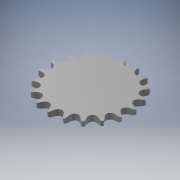
# Autodesk Inventor part: Kettenrad der Rollenkette1
Saved by Autodesk Inventor 2018 (Build 220112000, 112)
## iProperties
Created: 2018-01-11
Part Number: Kettenrad der Rollenkette1
Material: Steel
Document SubType Name: Modeling
Designer: Dominik
Density: 1 g/cm^3
Appearance: Steel
CustomPartVersion: 1
Author: Dominik
Autodesk Inventor part; units mm, degrees
ref_plane "YZ Plane" through (0, 0, 0) normal (1, 0, 0) x (0, 1, 0)
ref_plane "XZ Plane" through (0, 0, 0) normal (0, 1, 0) x (-1, 0, 0)
sketch "Theoretisches Zahnprofil" plane through (0, 0, 0) normal (0, 0, 1) x (1, 0, 0)
  circle A0 centre (0, 0) radius 38.5796 construction
  line L0 (0, 0) -> (0, 38.5796) construction
  line L1 (0, 0) -> (12.5268, 36.4893) construction
  circle A1 centre (0, 0) radius 41.8635
  arc A2 (-3.0854, 36.1554) -> (3.0854, 36.1554) centre (0, 38.5796) ccw
  line L2 (0, 38.5796) -> (12.5268, 36.4893) construction
  line L3 (0, 38.5796) -> (4.8877, 42.4201) construction
  line L4 (4.8877, 42.4201) -> (-4.4388, 38.441) construction
  arc A3 (6.2377, 41.3962) -> (4.8113, 39.3142) centre (10.7296, 36.7892) ccw
  arc A4 (-4.8113, 39.3142) -> (-6.2377, 41.3962) centre (-10.7296, 36.7892) ccw
  line L5 (-10.7296, 36.7892) -> (-4.8113, 39.3142) construction
  arc A5 (-4.4388, 38.441) -> (-3.0854, 36.1554) centre (4.8877, 42.4201) ccw
  line L6 (-4.4388, 38.441) -> (-4.8113, 39.3142)
  arc A6 (3.0854, 36.1554) -> (4.4388, 38.441) centre (-4.8877, 42.4201) ccw
  line L7 (4.8113, 39.3142) -> (4.4388, 38.441)
  line L8 (0, 0) -> (6.8905, 41.2925) construction
  point P0 (6.2634, 37.5345)
  dimension "d0" = 77.1593
  dimension "d2" = 18.947
  dimension "d3" = 3.9238
  dimension "d10" = 128.158
  dimension "d11" = 15.053
  dimension "d12" = 6.216
  dimension "d13" = 10.1398
  dimension "d14" = 10.878
  dimension "d23" = 3.81
  constraints: 18 end point, 15 point on circle, 7 centre point, 3 coincident, 3 point on line, 3 symmetric about line, 3 tangent, 1 equal radius, 1 midpoint, 1 parallel, 1 vertical, 1 other
  measures "d0" diameter of A0
  measures "d2" angle of L1 L0
  measures "d3" radius of A2
  measures "d10" angle of L3 L0
  measures "d11" angle of L4 L3
  measures "d12" distance of L2.start L3.end
  measures "d13" distance of L3.end L4.end
  measures "d14" distance of A3.centre L0.end
  measures "d23" distance from line of L8.end L2
sketch "Zahnprofil" plane through (0, 0, 0) normal (0, 0, 1) x (1, 0, 0)
  arc A0 (-3.6286, 37.0864) -> (3.6286, 37.0864) centre (0, 38.5796) ccw
  arc A1 (6.0969, 41.4171) -> (3.6286, 37.0864) centre (21.7357, 29.6348) ccw
  arc A2 (-3.6286, 37.0864) -> (-6.0969, 41.4171) centre (-21.7357, 29.6348) ccw
  line L0 (0, 0) -> (0, 38.5796) construction
  line L1 (0, 38.5796) -> (3.6286, 37.0864) construction
  line L2 (0, 38.5796) -> (-3.6286, 37.0864) construction
  circle A3 centre (0, 0) radius 41.8635 projected
  dimension "d44" = 135.263
  dimension "d45" = 19.5804
  dimension "d46" = 3.9238
  constraints: 9 point on circle, 6 end point, 3 centre point, 2 tangent, 1 coincident, 1 equal radius, 1 vertical, 1 other
  measures "d44" angle of L2 L1
  measures "d45" radius of A1
  measures "d46" radius of A0
sketch "Schnittprofil" plane through (0, 0, 0) normal (1, 0, 0) x (0, 1, 0)
  line L0 (41.8635, 0) -> (-41.8635, 0) projected
  line L1 (28.5923, 2.9063) -> (-28.5923, 2.9063)
  line L2 (-28.5923, 2.9063) -> (-28.5923, -2.9062)
  line L3 (-28.5923, -2.9062) -> (28.5923, -2.9062)
  line L4 (28.5923, -2.9062) -> (28.5923, 2.9063)
  line L5 (28.5923, 2.9062) -> (41.8635, 2.9062) construction
  line L6 (41.8635, 2.9062) -> (41.8635, -2.9062) construction
  line L7 (41.8635, -2.9062) -> (28.5923, -2.9062) construction
  line L8 (28.5923, -2.9062) -> (28.5923, 2.9062)
  arc A0 (41.8635, 2.1443) -> (37.5305, 2.9063) centre (37.5305, -9.7937) ccw
  arc A1 (37.5305, -2.9063) -> (41.8635, -2.1443) centre (37.5305, 9.7937) ccw
  line L9 (37.5305, 2.9063) -> (0, 2.9062)
  line L10 (0, 2.9062) -> (0, -2.9062)
  line L11 (0, -2.9062) -> (37.5305, -2.9063)
  line L12 (0, 2.9062) -> (0, -2.9062)
  line L13 (41.8635, 2.1443) -> (41.8635, -2.1443)
  point P0 (0, 0)
  point P1 (0, 0)
  dimension "d30" = 5.8125
  dimension "d31" = 57.1845
  dimension "d32" = 5.8125
  dimension "d33" = 0.762
  dimension "d34" = 12.7
  dimension "d43" = 2.9062
  constraints: 26 end point, 7 midpoint, 5 perpendicular, 4 parallel, 4 point on circle, 3 point on line, 3 symmetric about line, 2 centre point, 2 horizontal, 2 tangent, 1 collinear, 1 other
  measures "d30" distance between parallel lines of L7 L5
  measures "d31" distance between parallel lines of L2 L4
  measures "d32" distance between parallel lines of L3 L1
  measures "d33" distance from line of L13.start L5
  measures "d34" radius of A0
  measures "d43" distance between parallel lines of L3 L0
revolve "Ummantelung" add sketch "Schnittprofil" angle 360 about axis through (0, 0, 2.9062) along (0, 0, -1) contours L10 L3 L2 L0 | L0 L2 L1 L10
revolve "Reihe" add sketch "Schnittprofil" angle 360 about axis through (0, 0, 2.9062) along (0, 0, -1) contours L13 A1 L11 L4 L0 | L0 L4 L9 A0 L13 | L4 L3 L10 L0 | L0 L10 L1 L4
pattern_of_one "Reihenanordnung"
extrude "Theoretischer Zahn" cut sketch "Theoretisches Zahnprofil" along normal through all both and the other way through all contours A3 L7 A6 A2 A5 L6 A4 A1 picked at (0, 39.4262)
extrude "Zahn" [suppressed]
pattern_circular "Zahnanordnung" count 19 over 360 about axis through (0, 0, -10) along (0, 0, 1) of "Theoretischer Zahn"
ref_plane "Planungsebene" through (0, 38.5796, 0) normal (1, 0, 0) x (0, 1, 0)
equation "\"d3\" = 0.5 * da_Dr + da_SC"
equation "\"d12\" = 0.8 * da_Dr"
equation "\"d13\" = 1.3 * da_Dr + da_SC"
equation "\"d14\" = 1.4 * da_Dr"
equation "\"d23\" = da_Ha"
equation "\"d44\" = da_Alfa"
equation "\"d45\" = da_Re"
equation "\"d46\" = da_Ri"
equation "\"d30\" = da_Bf"
equation "\"d31\" = da_Ds"
equation "\"d32\" = da_Bs"
equation "\"d33\" = da_Ba"
equation "\"d34\" = da_Rx"
equation "\"d40\" = da_pt"
equation "\"form_type\" = 0"
equation "\"da_p\" = 12.7"
equation "\"da_Dr\" = 7.77"
equation "\"da_SC\" = 0.03885"
equation "\"da_Ha\" = 3.81"
equation "\"da_pt\" = 13.92"
equation "\"da_Bf\" = 5.8125"
equation "\"da_Ba\" = 0.762"
equation "\"da_Rx\" = 12.7"
equation "\"da_Ra\" = 0.508"
equation "\"da_Bs\" = 5.8125"
equation "\"da_Ds\" = 57.18453"
equation "\"da_Re\" = 19.5804"
equation "\"da_Ri\" = 3.92385"
equation "\"da_Alfa\" = 135.263deg"
body "Solid1"
